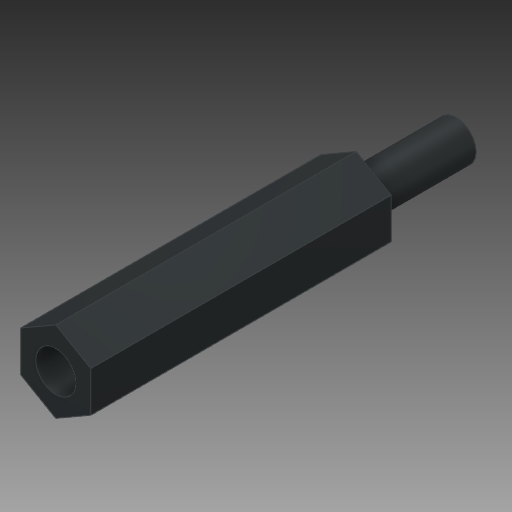
# Autodesk Inventor part: 六角スペーサー
Saved by Autodesk Inventor 2019 (Build 230136000, 136)
## iProperties
Created: 2020-09-27
Part Number: 六角スペーサー
Material: 鉄、ダクタイル鋳鉄
Document SubType Name: Modeling
Designer: Toshihito
Density: 7.15 g/cm^3
Appearance: 鉄 ねずみ鋳鉄
Mass: 8.88667 g
Surface Area: 10.9089 cm^2
Volume: 1.24289 cm^3
Author: Toshihito
Autodesk Inventor part; units mm, degrees
ref_plane "YZ Plane" through (0, 0, 0) normal (1, 0, 0) x (0, 1, 0)
ref_plane "XZ Plane" through (0, 0, 0) normal (0, 1, 0) x (-1, 0, 0)
ref_plane "XY Plane" through (0, 0, 0) normal (0, 0, 1) x (1, 0, 0)
sketch "スケッチ1" plane through (0, 0, 0) normal (0, 0, 1) x (1, 0, 0)
  circle A0 centre (0, 0) radius 3.5 construction
  line L0 (3.5, -2.0207) -> (0, -4.0415)
  line L1 (0, -4.0415) -> (-3.5, -2.0207)
  line L2 (-3.5, -2.0207) -> (-3.5, 2.0207)
  line L3 (-3.5, 2.0207) -> (0, 4.0415)
  line L4 (0, 4.0415) -> (3.5, 2.0207)
  line L5 (3.5, 2.0207) -> (3.5, -2.0207)
  point P0 (3.5, 0)
  dimension "d0" = 7
  constraints: 12 end point, 2 coincident, 1 horizontal alignment, 1 midpoint, 15 other
extrude "押し出し1" add sketch "スケッチ1" along normal blind 30
sketch "スケッチ2" plane through (0, 0, 30) normal (0, 0, 1) x (1, 0, 0)
  point P0 (0, 0)
  point P1 (0, 0)
  constraints: 1 coincident
hole "穴1" at (0, 0, 30) direction (0, 0, -1) diameter 4 depth 12 tip angle 118
sketch "スケッチ3" plane through (0, 0, 0) normal (0, 0, -1) x (-1, 0, 0)
  circle A0 centre (0, 0) radius 2
  dimension "d10" = 4
  constraints: 1 centre point, 1 coincident
  measures "d10" diameter of A0
extrude "押し出し2" add sketch "スケッチ3" along normal blind 10
